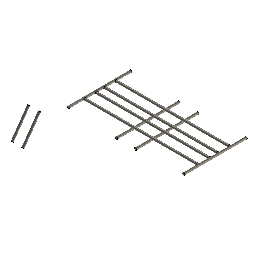
Kerbecs (Autodesk Fusion 360 design; units mm, degrees)
Autodesk Fusion 360 part; units mm, degrees
cylinder "CylinderPrimitive3" add diameter 18 height 736 placed x (0, 0, -1) y (0, 1, 0) z (1, 0, 0) at (0, 0, 0) makes body 1
copy_body "CopyPasteBodies4" bodies 1 makes body 2
move_body "Move2" bodies 2 to x (1, 0, 0) y (0, 1, 0) z (0, 0, 1) at (0, 218, 0)
copy_body "CopyPasteBodies5" bodies 1 2 makes body 3 makes body 4
move_body "Move3" bodies 3 to x (1, 0, 0) y (0, 1, 0) z (0, 0, 1) at (0, 79, 0)
move_body "Move4" bodies 4 to x (1, 0, 0) y (0, 1, 0) z (0, 0, 1) at (0, -79, 0)
cylinder "CylinderPrimitive4" add diameter 18 height 436 placed x (1, 0, 0) y (0, 0, -1) z (0, 1, 0) at (0, 0, 25) separate body makes body 5
move_body "Move5" bodies 5 to x (1, 0, 0) y (0, 1, 0) z (0, 0, 1) at (0, -109, 0)
move_body "Move6" bodies 5 to x (1, 0, 0) y (0, 1, 0) z (0, 0, 1) at (0, 0, -7)
move_body "Move7" bodies 5 to x (1, 0, 0) y (0, 1, 0) z (0, 0, 1) at (9, 0, 0)
copy_body "CopyPasteBodies6" bodies 5 makes body 6
move_body "Move8" bodies 6 to x (1, 0, 0) y (0, 1, 0) z (0, 0, 1) at (318, 0, 0)
copy_body "CopyPasteBodies7" bodies 6 makes body 7
move_body "Move9" bodies 7 to x (1, 0, 0) y (0, 1, 0) z (0, 0, 1) at (132, 0, 0)
copy_body "CopyPasteBodies8" bodies 7 makes body 8
move_body "Move10" bodies 8 to x (1, 0, 0) y (0, 1, 0) z (0, 0, 1) at (318, 0, 0)
move_face "OffsetFaces1" offset 50 1 faces at (736, 0.3267, 5.1676) on bodies 1
move_face "OffsetFaces2" offset 50 1 faces at (736, 79.3267, 5.1676) on bodies 3
move_face "OffsetFaces3" offset 50 1 faces at (736, 141.3455, -1.8705) on bodies 4
move_face "OffsetFaces4" offset 50 1 faces at (736, 220.3455, -1.8705) on bodies 2
move_body "Move11" bodies 5 to x (1, 0, 0) y (0, 1, 0) z (0, 0, 1) at (-18, 0, 0)
move_body "Move12" bodies 5 to x (1, 0, 0) y (0, 1, 0) z (0, 0, 1) at (0, 0, -18)
move_body "Move13" bodies 8 to x (1, 0, 0) y (0, 1, 0) z (0, 0, 1) at (18, 0, -18)
move_body "Move14" bodies 6 7 to x (1, 0, 0) y (0, 1, 0) z (0, 0, 1) at (0, 0, -36)
cylinder "CylinderPrimitive5" add diameter 18 height 200 placed x (1, 0, 0) y (0, 0, -1) z (0, 1, 0) at (0, 0, -75) separate body makes body 9
move_body "Move16" bodies 9 to x (1, 0, 0) y (0, 1, 0) z (0, 0, 1) at (0, -500, 0)
move_body "Move17" bodies 9 to x (1, 0, 0) y (0, 1, 0) z (0, 0, 1) at (0, 0, 75)
move_body "Move18" bodies 9 to x (1, 0, 0) y (0, 0.573576, 0.819152) z (0, -0.819152, 0.573576) at (0, -220.5842, 405.7382)
copy_body "CopyPasteBodies10" bodies 9 makes body 10
move_body "Move19" bodies 10 to x (1, 0, 0) y (0, 1, 0) z (0, 0, 1) at (75, 0, 0)
cylinderprimitive "CylinderPrimitive2" [suppressed]
equation "d11 = 18.00 mm + 200 mm"
equation "d14 = ( ( 18 + 200 ) / 2 ) * 1 mm - 30 mm"
equation "d17 = -( ( ( 18 + 200 ) / 2 ) * 1 mm - 30 mm )"
equation "d33 = 114 mm + 18 mm"
named bodies: "Pipe 1", "Pipe 4", "Pipe 1 (1)", "Pipe 1 (1) (1)", "Pipe 2", "Pipe 3", "Pipe 5", "Pipe 6", "Pipe 5 (1)", "Pipe 7", "Pipe 5 (1) (1)", "Pipe8", "Thigh 1", "Thigh 2"
